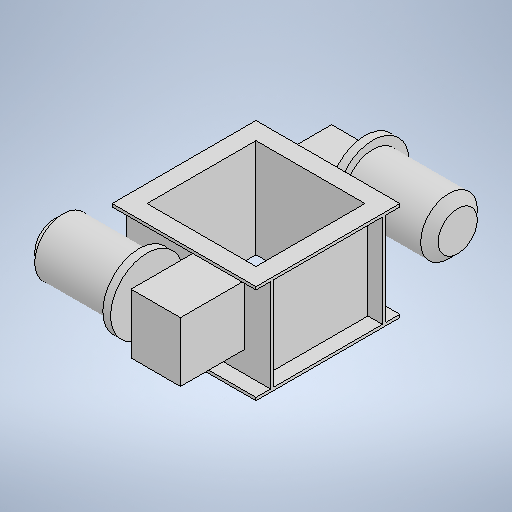
# Autodesk Inventor part: Измельчитель комков
Saved by Autodesk Inventor 2025 (Build 290162010, 162A)
## iProperties
Created: 2024-10-30
Part Number: Измельчитель комков
Material: Generic
Document SubType Name: Modeling
Designer: pokla
Density: 1 g/cm^3
Appearance: Default
Author: pokla
Autodesk Inventor part; units mm, degrees
ref_plane "YZ Plane" through (0, 0, 0) normal (1, 0, 0) x (0, 1, 0)
ref_plane "XZ Plane" through (0, 0, 0) normal (0, 1, 0) x (-1, 0, 0)
ref_plane "XY Plane" through (0, 0, 0) normal (0, 0, 1) x (1, 0, 0)
sketch "Sketch1" plane through (0, 0, 0) normal (0, 0, 1) x (1, 0, 0)
  line L0 (-247.5, 247.5) -> (247.5, 247.5)
  line L1 (247.5, 247.5) -> (247.5, -247.5)
  line L2 (247.5, -247.5) -> (-247.5, -247.5)
  line L3 (-247.5, -247.5) -> (-247.5, 247.5)
  line L4 (-247.5, -247.5) -> (247.5, 247.5) construction
  point P0 (0, 0)
  point P1 (0, 0)
  dimension "d0" = 495
  dimension "d1" = 495
  constraints: 10 end point, 2 parallel, 1 coincident, 1 horizontal, 1 midpoint, 1 perpendicular
  measures "d0" distance of L0.start L0.end
  measures "d1" distance of L2.end L0.start
extrude "Extrusion1" add sketch "Sketch1" against normal blind 10
sketch "Sketch2" plane through (0, 0, -10) normal (0, 0, -1) x (-1, 0, 0)
  line L0 (197.5, -197.5) -> (-197.5, -197.5)
  line L1 (-197.5, -197.5) -> (-197.5, 197.5)
  line L2 (-197.5, 197.5) -> (197.5, 197.5)
  line L3 (197.5, 197.5) -> (197.5, -197.5)
  line L4 (197.5, -197.5) -> (-197.5, 197.5) construction
  line L5 (247.5, -247.5) -> (247.5, 247.5) projected
  line L6 (197.5, -197.5) -> (247.5, -197.5)
  line L7 (247.5, -197.5) -> (247.5, -187.5)
  line L8 (247.5, -187.5) -> (197.5, -187.5)
  line L9 (197.5, -187.5) -> (197.5, -197.5)
  line L10 (197.5, 197.5) -> (247.5, 197.5)
  line L11 (247.5, 197.5) -> (247.5, 187.5)
  line L12 (247.5, 187.5) -> (197.5, 187.5)
  line L13 (197.5, 187.5) -> (197.5, 197.5)
  line L14 (-247.5, 247.5) -> (-247.5, -247.5) projected
  line L15 (-197.5, -197.5) -> (-247.5, -197.5)
  line L16 (-247.5, -197.5) -> (-247.5, -187.5)
  line L17 (-247.5, -187.5) -> (-197.5, -187.5)
  line L18 (-197.5, -187.5) -> (-197.5, -197.5)
  line L19 (-197.5, 197.5) -> (-247.5, 197.5)
  line L20 (-247.5, 197.5) -> (-247.5, 187.5)
  line L21 (-247.5, 187.5) -> (-197.5, 187.5)
  line L22 (-197.5, 187.5) -> (-197.5, 197.5)
  point P0 (0, 0)
  point P1 (0, 0)
  dimension "d4" = 395
  dimension "d5" = 395
  dimension "d19" = 10
  dimension "d20" = 10
  dimension "d21" = 10
  dimension "d22" = 10
  constraints: 42 end point, 10 parallel, 5 horizontal, 5 perpendicular, 4 point on line, 1 coincident, 1 midpoint
  measures "d4" distance of L0.start L0.end
  measures "d5" distance of L2.end L0.start
  measures "d19" distance between parallel lines of L6 L8
  measures "d20" distance between parallel lines of L10 L12
  measures "d21" distance between parallel lines of L17 L15
  measures "d22" distance between parallel lines of L21 L19
extrude "Extrusion2" add sketch "Sketch2" along normal blind 320 contours L0 L1 L2 L3 | L3 L8 L5 L6 | L15 L14 L17 L1 | L3 L10 L5 L12 | L21 L14 L19 L1
sketch "Sketch3" plane through (0, 0, -330) normal (0, 0, -1) x (-1, 0, 0)
  line L0 (-247.5, -247.5) -> (247.5, -247.5)
  line L1 (247.5, -247.5) -> (247.5, 247.5)
  line L2 (247.5, 247.5) -> (-247.5, 247.5)
  line L3 (-247.5, 247.5) -> (-247.5, -247.5)
  line L4 (-247.5, -247.5) -> (247.5, 247.5) construction
  point P0 (0, 0)
  point P1 (0, 0)
  dimension "d8" = 495
  dimension "d9" = 495
  constraints: 10 end point, 2 parallel, 1 coincident, 1 horizontal, 1 midpoint, 1 perpendicular
  measures "d8" distance of L2.end L0.start
  measures "d9" distance of L0.start L0.end
extrude "Extrusion3" add sketch "Sketch3" along normal blind 10
sketch "Sketch4" plane through (0, 0, 0) normal (0, 0, 1) x (1, 0, 0)
  line L0 (-187.5, -187.5) -> (187.5, -187.5)
  line L1 (187.5, -187.5) -> (187.5, 187.5)
  line L2 (187.5, 187.5) -> (-187.5, 187.5)
  line L3 (-187.5, 187.5) -> (-187.5, -187.5)
  line L4 (-187.5, -187.5) -> (187.5, 187.5) construction
  point P0 (0, 0)
  point P1 (0, 0)
  dimension "d12" = 375
  dimension "d13" = 375
  constraints: 10 end point, 2 parallel, 1 coincident, 1 horizontal, 1 midpoint, 1 perpendicular
  measures "d12" distance of L2.end L0.start
  measures "d13" distance of L0.start L0.end
extrude "Extrusion4" cut sketch "Sketch4" against normal through all
sketch "Sketch6" plane through (-247.5, -197.5, -10) normal (0, -1, 0) x (1, 0, 0)
  line L0 (235, -42.5) -> (405, -42.5)
  line L1 (405, -42.5) -> (405, -247.5)
  line L2 (405, -247.5) -> (235, -247.5)
  line L3 (235, -247.5) -> (235, -42.5)
  line L4 (235, -42.5) -> (405, -247.5) construction
  line L5 (495, 0) -> (495, -320) projected
  line L6 (495, -330) -> (0, -330) projected
  point P0 (247.5, 10)
  point P1 (320, -145)
  dimension "d23" = 205
  dimension "d24" = 170
  dimension "d25" = 175
  dimension "d26" = 185
  constraints: 10 end point, 2 parallel, 1 horizontal, 1 midpoint, 1 perpendicular
  measures "d23" distance of L2.end L0.start
  measures "d24" distance of L0.start L0.end
  measures "d25" distance from line of point (320, -145) L5
  measures "d26" distance from line of L6 point (320, -145)
extrude "Extrusion5" add sketch "Sketch6" along normal blind 220
sketch "Sketch7" plane through (-12.5, -197.5, -257.5) normal (-1, 0, 0) x (0, 0, 1)
  circle A0 centre (160, -165) radius 125
  line L0 (205, 0) -> (205, -220) projected
  line L1 (205, -220) -> (0, -220) projected
  point P0 (257.5, 197.5)
  dimension "d5" = 395
  dimension "d30" = 250
  dimension "d33" = 45
  dimension "d34" = 55
  constraints: 1 centre point
  measures "d30" diameter of A0
  measures "d33" distance from line of L0 A0.centre
  measures "d34" distance from line of L1 A0.centre
extrude "Extrusion6" add sketch "Sketch7" along normal blind 27
sketch "Sketch8" plane through (-39.5, -362.5, -97.5) normal (-1, 0, 0) x (0, 0, 1)
  circle A0 centre (0, 0) radius 97.5
  circle A1 centre (0, 0) radius 125 projected
  point P0 (97.5, 362.5)
  dimension "d37" = 195
  constraints: 1 centre point, 1 coincident
  measures "d37" diameter of A0
extrude "Extrusion7" add sketch "Sketch8" along normal blind 292 contours A0
pattern_circular "Circular Pattern1" count 2 over 360 about axis through (0, 0, -10) along (0, 0, 1) of "Extrusion7", "Extrusion6", "Extrusion5"
sketch "Sketch10" plane through (-197.5, -187.5, -10) normal (-1, 0, 0) x (0, 0, 1)
  line L0 (-77.5, 363.5) -> (-242.5, 363.5)
  line L1 (-242.5, 363.5) -> (-242.5, 276.5)
  line L2 (-242.5, 276.5) -> (-77.5, 276.5)
  line L3 (-77.5, 276.5) -> (-77.5, 363.5)
  line L4 (0, 375) -> (-320, 375) projected
  point P0 (10, 187.5)
  point P1 (-77.5, 320)
  point P2 (-160, 363.5)
  point P3 (-160, 375)
  dimension "d44" = 165
  dimension "d45" = 87
  dimension "d46" = 55
  constraints: 8 end point, 3 midpoint, 2 parallel, 1 horizontal, 1 perpendicular, 1 vertical alignment
  measures "d44" distance of L1.end L2.end
  measures "d45" distance of L2.end L0.start
  measures "d46" distance from line of L4 point (-77.5, 320)
extrude "Extrusion8" add sketch "Sketch10" along normal blind 125
chamfer "Chamfer1" distance 30 angle 45 2 edges at (-322.5, 132.5, -87.5) (-322.5, 132.5, -252.5)
chamfer "Chamfer2" distance 30 angle 45 2 edges at (331.5, 362.5, -195) (-331.5, -362.5, -195)
equation "\"d1\" = d0"
equation "\"d5\" = d4"
equation "\"d20\" = d19"
equation "\"d21\" = d19"
equation "\"d22\" = d19"
equation "\"d8\" = d0"
equation "\"d9\" = d8"
body "Solid1"
